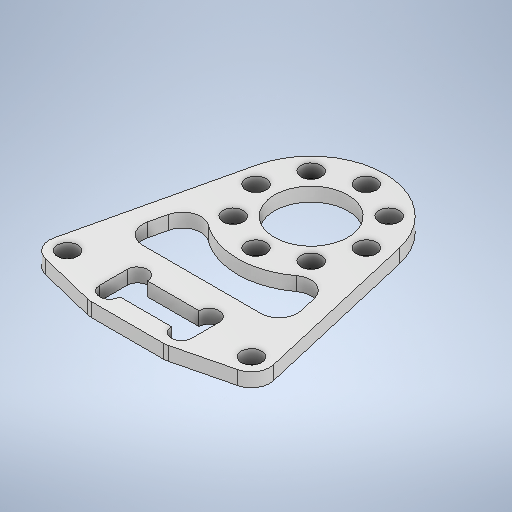
# Autodesk Inventor part: kata
Saved by Autodesk Inventor 2025.1 (Build 291241000, 241)
## iProperties
Created: 2024-09-04
Part Number: kata
Material: アルミニウム 2014-T4
Document SubType Name: Modeling
Designer: right
Density: 2.8 g/cm^3
Appearance: サテン
Mass: 1.25351 g
Surface Area: 9.76459 cm^2
Volume: 0.447683 cm^3
Author: right
Autodesk Inventor part; units mm, degrees
ref_plane "YZ Plane" through (0, 0, 0) normal (1, 0, 0) x (0, 1, 0)
ref_plane "XZ Plane" through (0, 0, 0) normal (0, 1, 0) x (-1, 0, 0)
ref_plane "XY Plane" through (0, 0, 0) normal (0, 0, 1) x (1, 0, 0)
sketch "スケッチ1" plane through (0, 0, 0) normal (0, 1, 0) x (-1, 0, 0)
  circle A0 centre (0, 0) radius 4
  circle A1 centre (0, 0) radius 6 construction
  circle A2 centre (0, 0) radius 8
  circle A3 centre (0, -6) radius 1.1
  circle A4 centre (4.2426, -4.2426) radius 1.1
  circle A5 centre (6, 0) radius 1.1
  circle A6 centre (4.2426, 4.2426) radius 1.1
  circle A7 centre (0, 6) radius 1.1
  circle A8 centre (-4.2426, 4.2426) radius 1.1
  circle A9 centre (-6, 0) radius 1.1
  circle A10 centre (-4.2426, -4.2426) radius 1.1
  line L0 (5, 15) -> (-5, 15)
  line L1 (-5, 15) -> (-5, 18)
  line L2 (-5, 18) -> (5, 18)
  line L3 (5, 18) -> (5, 15)
  circle A11 centre (3.9, 15) radius 1.1
  line L4 (0, 15) -> (0, 18) construction
  circle A12 centre (-3.9, 15) radius 1.1
  line L5 (-5, 16.5) -> (5, 16.5) construction
  circle A13 centre (3.9, 18) radius 1.1
  circle A14 centre (-3.9, 18) radius 1.1
  circle A15 centre (-10, 16.5) radius 1.1
  circle A16 centre (10, 16.5) radius 1.1
  circle A17 centre (10, 16.5) radius 2
  circle A18 centre (3.9, 18) radius 2
  circle A19 centre (-10, 16.5) radius 2
  line L6 (7.7918, -1.8132) -> (11.948, 16.0467)
  line L7 (-7.7918, -1.8132) -> (-11.948, 16.0467)
  line L8 (10.4776, 18.4421) -> (4.3776, 19.9421)
  circle A20 centre (-3.9, 18) radius 2
  line L9 (-10.4776, 18.4421) -> (-4.3776, 19.9421)
  line L10 (3.9, 20) -> (-4.1423, 20)
  point P0 (2.8, 18)
  point P1 (5, 18)
  point P2 (2.8, 15)
  point P3 (-2.8, 15)
  point P4 (-5, 15)
  point P5 (-5, 18)
  point P6 (-2.8, 18)
  point P7 (-3.9, 20)
  point P8 (-10.4776, 18.4421)
  dimension "d1" = 12
  dimension "d11" = 2.2
  dimension "d16" = 4
  dimension "d0" = 8
  dimension "d2" = 16
  dimension "d3" = 2.2
  dimension "d6" = 360
  dimension "d8" = 10
  dimension "d9" = 3
  dimension "d10" = 15
  dimension "d12" = 2.2
  dimension "d13" = 5
  dimension "d14" = 4
  dimension "d15" = 4
  constraints: 22 end point, 17 centre point, 7 symmetric about line, 6 coincident, 6 point on circle, 6 tangent, 4 midpoint, 3 vertical alignment, 2 horizontal, 2 parallel, 2 perpendicular, 2 point on line, 1 horizontal alignment, 34 other
  measures "d0" diameter of A0
  measures "d2" diameter of A2
  measures "d3" diameter of A3
  measures "d8" distance of L0.start L0.end
  measures "d9" distance of L2.end L0.start
  measures "d10" distance of L4.start point (0, 0)
  measures "d12" diameter of A15
  measures "d13" distance from line of L1 A15.centre
  measures "d14" diameter of A17
  measures "d15" diameter of A18
extrude "押し出し1" add sketch "スケッチ1" along normal blind 1.5 contours A2 | A2 L7 A19 L9 A20 L1 A12 L0 A11 L3 A18 L8 A17 L6 | A19 | A17 | A20 L2 A14 L1 | A18 L3 A13 L2 | L10 A18 L2 A20
sketch "スケッチ2" plane through (0, 1.5, 0) normal (0, 1, 0) x (1, 0, 0)
  line L0 (-8.9295, -11.9) -> (8.9295, -11.9)
  line L1 (8.9295, -11.9) -> (7.0432, -3.7939)
  line L2 (-7.7918, 1.8132) -> (-11.948, -16.0467) projected
  circle A0 centre (0, 0) radius 8
  line L3 (-8.9295, -11.9) -> (-7.0432, -3.7939)
  line L4 (-7.7918, 1.8132) -> (-11.948, -16.0467) projected
  line L5 (11.948, -16.0467) -> (7.7918, 1.8132) projected
  arc A1 (-2.8, -15) -> (-5, -15) centre (-3.9, -15) ccw projected
  point P0 (-3.9, -13.9)
  dimension "d19" = 2
  dimension "d20" = 2
  dimension "d21" = 2
  constraints: 6 end point, 4 point on circle, 2 parallel, 1 centre point, 1 coincident, 1 horizontal
  measures "d19" distance between parallel lines of L2 L3
  measures "d20" distance from line of point (-3.9, -13.9) L0
  measures "d21" distance between parallel lines of L5 L1
extrude "押し出し2" cut sketch "スケッチ2" against normal through all contours L3 A0 L1 L0
fillet "フィレット1" radius 2 4 edges at (-7.0432, 0.75, 3.7939) (7.0432, 0.75, 3.7939) (8.9295, 0.75, 11.9) (-8.9295, 0.75, 11.9)
equation "\"d21\" = d19"
